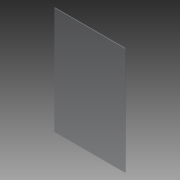
# Autodesk Inventor part: pneumatics board 1
Saved by Autodesk Inventor 2014 (Build 180170000, 170)
## iProperties
Created: 2014-01-20
Part Number: pneumatics board 1
Material: Polycarbonate, Clear
Document SubType Name: Modeling
Designer: Arpan
Density: 1.2 g/cm^3
Appearance: Polycarbonate - Clear
Author: Arpan
Autodesk Inventor part; units mm, degrees
ref_plane "YZ Plane" through (0, 0, 0) normal (1, 0, 0) x (0, 1, 0)
ref_plane "XZ Plane" through (0, 0, 0) normal (0, 1, 0) x (-1, 0, 0)
ref_plane "XY Plane" through (0, 0, 0) normal (0, 0, 1) x (1, 0, 0)
sketch "Sketch1" plane through (0, 0, 0) normal (0, 0, 1) x (1, 0, 0)
  line L0 (0, 0) -> (-150.114, 0)
  line L1 (0, 228.6) -> (0, 0)
  line L2 (0, 228.6) -> (-150.114, 228.6)
  line L3 (-150.114, 228.6) -> (-150.114, 0)
  dimension "d8" = 150.114
  dimension "d28" = 228.6
  constraints: 8 end point, 2 perpendicular, 1 horizontal
  measures "d8" distance of L0.start L0.end
  measures "d28" distance between parallel lines of L0 L2
extrude "Extrusion1" add sketch "Sketch1" along normal blind 1.5875
body "Solid1"
